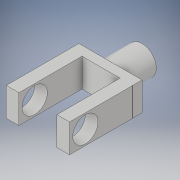
# Autodesk Inventor part: Connector
Saved by Autodesk Inventor 2019 (Build 230136000, 136)
## iProperties
Created: 2021-10-31
Part Number: Connector
Material: Generic
Document SubType Name: Modeling
Designer: Mohamed Teleb
Density: 1 g/cm^3
Appearance: Default
Author: Mohamed Teleb
Autodesk Inventor part; units mm, degrees
ref_plane "YZ Plane" through (0, 0, 0) normal (1, 0, 0) x (0, 1, 0)
ref_plane "XZ Plane" through (0, 0, 0) normal (0, 1, 0) x (-1, 0, 0)
ref_plane "XY Plane" through (0, 0, 0) normal (0, 0, 1) x (1, 0, 0)
sketch "Sketch1" plane through (0, 0, 0) normal (0, 0, 1) x (1, 0, 0)
  circle A0 centre (0, 0) radius 2.75
  circle A1 centre (0, 0) radius 4.5
  dimension "d0" = 5.5
  dimension "d1" = 9
  constraints: 2 centre point, 2 coincident
  measures "d0" diameter of A0
  measures "d1" diameter of A1
extrude "Extrusion1" add sketch "Sketch1" along normal blind 10
sketch "Sketch2" plane through (0, 0, 10) normal (0, 0, 1) x (1, 0, 0)
  line L0 (-10, 4.5) -> (10, 4.5)
  line L1 (10, 4.5) -> (10, -4.5)
  line L2 (10, -4.5) -> (-10, -4.5)
  line L3 (-10, -4.5) -> (-10, 4.5)
  point P0 (0, 0)
  dimension "d4" = 20
  dimension "d5" = 10
  constraints: 8 end point, 2 parallel, 1 horizontal, 1 perpendicular
  measures "d4" distance of L1.end L2.end
  measures "d5" distance from line of L3 point (0, 0)
extrude "Extrusion2" add sketch "Sketch2" along normal blind 3
sketch "Sketch3" plane through (0, 0, 13) normal (0, 0, 1) x (1, 0, 0)
  line L0 (10, 4.5) -> (-10, 4.5) projected
  line L1 (-10, -4.5) -> (10, -4.5) projected
  line L2 (-10, 4.5) -> (-6, 4.5)
  line L3 (-6, 4.5) -> (-6, -4.5)
  line L4 (-6, -4.5) -> (-10, -4.5)
  line L5 (-10, -4.5) -> (-10, 4.5)
  line L6 (10.0384, 4.5) -> (6.0384, 4.5)
  line L7 (6.0384, 4.5) -> (6.0384, -4.5)
  line L8 (6.0384, -4.5) -> (10.0384, -4.5)
  line L9 (10.0384, -4.5) -> (10.0384, 4.5)
  point P0 (0, 0)
  dimension "d8" = 4
  dimension "d9" = 4
  constraints: 16 end point, 4 parallel, 3 point on line, 2 horizontal, 2 perpendicular
  measures "d8" distance of L3.end L4.end
  measures "d9" distance of L8.end L7.end
extrude "Extrusion3" add sketch "Sketch3" along normal blind 20 contours L6 L9 L8 L1 L7 L0 | L3 L1 L5 L0
sketch "Sketch4" plane through (10.0384, -4.5, 13) normal (1, 0, 0) x (0, 0, -1)
  circle A0 centre (-15, 4.5) radius 4
  point P0 (13, 4.5)
  dimension "d12" = 8
  dimension "d13" = 28
  constraints: 1 centre point
  measures "d12" diameter of A0
  measures "d13" distance of point (13, 4.5) A0.centre
extrude "Extrusion4" cut sketch "Sketch4" against normal blind 27
body "Solid1"
